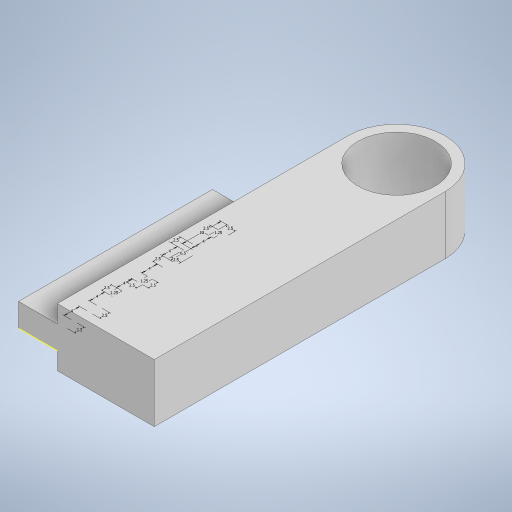
# Autodesk Inventor part: Part10
Saved by Autodesk Inventor 2023 (Build 270158000, 158)
## iProperties
Created: 2024-11-26
Part Number: Part10
Material: Generic
Document SubType Name: Modeling
Designer: 1ZHUSAM
Density: 1 g/cm^3
Appearance: Default
Author: 1ZHUSAM
Autodesk Inventor part; units mm, degrees
ref_plane "YZ Plane" through (0, 0, 0) normal (1, 0, 0) x (0, 1, 0)
ref_plane "XZ Plane" through (0, 0, 0) normal (0, 1, 0) x (-1, 0, 0)
ref_plane "XY Plane" through (0, 0, 0) normal (0, 0, 1) x (1, 0, 0)
sketch "Sketch1" plane through (0, 0, 0) normal (0, 1, 0) x (-1, 0, 0)
  circle A0 centre (0, 0) radius 10
  circle A1 centre (0, 0) radius 12.5
  line L0 (12.5, 0) -> (12.5, 50)
  line L1 (-12.5, 0) -> (-12.5, 50)
  line L2 (-12.5, 50) -> (12.5, 50)
  dimension "d0" = 20
  dimension "d1" = 25
  dimension "d2" = 50
  constraints: 6 end point, 2 centre point, 2 coincident, 2 point on circle, 2 tangent, 2 vertical, 1 perpendicular
  measures "d0" diameter of A0
  measures "d1" diameter of A1
  measures "d2" distance of L0.start L0.end
extrude "Extrusion1" add sketch "Sketch1" along normal blind 15
sketch "Sketch2" plane through (-12.5, 0, 0) normal (-1, 0, 0) x (0, 0, 1)
  line L0 (-12.5, 0) -> (-12.5, 15) projected
  line L1 (-12.5, 7.5) -> (37.5, 7.5)
  line L2 (25, 7.5) -> (25, 4.5)
  line L3 (25, 4.5) -> (25, 10.5)
  line L4 (25, 10.5) -> (75, 10.5)
  line L5 (75, 10.5) -> (75, 4.5)
  line L6 (75, 4.5) -> (25, 4.5)
  point P0 (0, 0)
  dimension "d5" = 50
  dimension "d8" = 3
  dimension "d9" = 6
  dimension "d10" = 50
  constraints: 12 end point, 3 perpendicular, 2 horizontal, 2 point on line, 1 midpoint
  measures "d5" distance of L1.start L1.end
  measures "d8" distance of L2.start L2.end
  measures "d9" distance of L2.end L3.end
  measures "d10" distance of L3.end L4.end
extrude "Extrusion2" add sketch "Sketch2" along normal blind 10
sketch "Sketch3" plane through (-12.5, 0, 50) normal (0, 0, 1) x (1, 0, 0)
  point P0 (12.5, 0)
sketch "Sketch4" plane through (-12.5, 0, 50) normal (0, 0, 1) x (1, 0, 0)
  line L0 (25, 0) -> (25, 15) projected
  line L1 (25, 0) -> (25, 15)
  line L2 (0, 15) -> (25, 15) projected
  line L3 (25, 15) -> (0, 15)
  line L4 (0, 0) -> (0, 15) projected
  line L5 (0, 15) -> (0, 0)
  line L6 (0, 0) -> (25, 0) projected
  line L7 (0, 0) -> (25, 0)
  point P0 (12.5, 0)
  constraints: 8 end point, 4 collinear
extrude "Extrusion3" add sketch "Sketch4" along normal blind 25
sketch "Sketch5" plane through (-12.5, 4.5, 25) normal (0, -1, 0) x (1, 0, 0)
  point P0 (12.5, -25)
sketch "Sketch6" plane through (-12.5, 4.5, 25) normal (0, -1, 0) x (1, 0, 0)
  line L0 (0, 0) -> (-10, 0) projected
  line L1 (-5, 0) -> (-5, 50)
  line L2 (0, 50) -> (-10, 50) projected
  line L3 (-5, 0) -> (-5, 10)
  line L4 (-3.75, 8.75) -> (-6.25, 8.75)
  line L5 (-6.25, 8.75) -> (-6.25, 11.25)
  line L6 (-6.25, 11.25) -> (-3.75, 11.25)
  line L7 (-3.75, 11.25) -> (-3.75, 8.75)
  line L8 (-3.75, 8.75) -> (-6.25, 11.25) construction
  line L9 (-6.25, 8.75) -> (-3.75, 11.25) construction
  line L10 (-5, 11.25) -> (-5, 15.25)
  line L11 (-3.75, 15.25) -> (-6.25, 15.25)
  line L12 (-6.25, 15.25) -> (-6.25, 17.75)
  line L13 (-6.25, 17.75) -> (-3.75, 17.75)
  line L14 (-3.75, 17.75) -> (-3.75, 15.25)
  point P0 (12.5, -25)
  dimension "d15" = 10
  dimension "d16" = 2.5
  dimension "d17" = 2.5
  dimension "d18" = 4
  dimension "d19" = 2.5
  constraints: 26 end point, 5 midpoint, 4 parallel, 2 horizontal, 2 perpendicular, 2 point on line
  measures "d15" distance of L1.start L3.end
  measures "d16" distance of L5.end L6.end
  measures "d17" distance of L4.end L5.end
  measures "d18" distance of L10.start L10.end
  measures "d19" distance of L11.end L12.end
sketch "Sketch7" plane through (-12.5, 4.5, 25) normal (0, -1, 0) x (1, 0, 0)
  line L0 (-4.9925, 17.7874) -> (-4.9925, 21.7874)
  line L1 (-4.9925, 21.7874) -> (-3.7425, 21.7874)
  line L2 (-3.7425, 21.7874) -> (-3.7425, 24.2874)
  line L3 (-3.7425, 24.2874) -> (-6.2425, 24.2874)
  line L4 (-6.2425, 24.2874) -> (-6.2425, 21.7874)
  line L5 (-6.2425, 21.7874) -> (-4.9925, 21.7874)
  line L6 (-4.9925, 24.2874) -> (-4.9925, 28.2874)
  line L7 (-4.9925, 28.2874) -> (-6.2425, 28.2874)
  line L8 (-6.2425, 28.2874) -> (-6.2425, 30.7874)
  line L9 (-6.2425, 30.7874) -> (-3.7425, 30.7874)
  line L10 (-3.7425, 30.7874) -> (-3.7425, 28.2874)
  line L11 (-4.9925, 28.2874) -> (-3.7425, 28.2874)
  line L12 (-4.9925, 30.7874) -> (-4.9925, 34.7874)
  line L13 (-4.9925, 34.7874) -> (-3.7425, 34.7874)
  line L14 (-3.7425, 34.7874) -> (-3.7425, 37.2874)
  line L15 (-3.7425, 37.2874) -> (-6.2425, 37.2874)
  line L16 (-6.2425, 37.2874) -> (-6.2425, 34.7874)
  line L17 (-6.2425, 34.7874) -> (-4.9925, 34.7874)
  line L18 (-4.9925, 37.2874) -> (-4.9925, 41.2874)
  line L19 (-4.9925, 41.2874) -> (-3.7425, 41.2874)
  line L20 (-3.7425, 41.2874) -> (-3.7425, 43.7874)
  line L21 (-3.7425, 43.7874) -> (-6.2425, 43.7874)
  line L22 (-6.2425, 43.7874) -> (-6.2425, 41.2874)
  line L23 (-6.2425, 41.2874) -> (-4.9925, 41.2874)
  line L24 (-5, 15.2622) -> (-5, 8.7622)
  line L25 (-5, 8.7622) -> (-5, 4.7622)
  line L26 (-5, 4.7622) -> (-6.25, 4.7622)
  line L27 (-6.25, 4.7622) -> (-6.25, 2.2622)
  line L28 (-6.25, 2.2622) -> (-3.75, 2.2622)
  line L29 (-3.75, 2.2622) -> (-3.75, 4.7622)
  line L30 (-3.75, 4.7622) -> (-5, 4.7622)
  point P0 (12.5, -25)
  dimension "d20" = 4
  dimension "d21" = 1.25
  dimension "d22" = 2.5
  dimension "d23" = 2.5
  dimension "d24" = 4
  dimension "d25" = 1.25
  dimension "d26" = 2.5
  dimension "d27" = 4
  dimension "d28" = 2.5
  dimension "d29" = 4
  dimension "d30" = 2.5
  dimension "d31" = 6.5
  dimension "d32" = 4
  dimension "d33" = 1.25
  dimension "d34" = 2.5
  dimension "d35" = 2.5
  constraints: 62 end point, 18 perpendicular, 11 point on line, 4 vertical, 3 midpoint, 2 horizontal, 1 collinear
  measures "d20" distance of L0.start L0.end
  measures "d21" distance of L0.end L1.end
  measures "d22" distance of L1.end L2.end
  measures "d23" distance of L2.end L3.end
  measures "d24" distance of L6.start L6.end
  measures "d25" distance of L6.end L7.end
  measures "d26" distance of L7.end L8.end
  measures "d27" distance of L12.start L12.end
  measures "d28" distance of L13.end L14.end
  measures "d29" distance of L18.start L18.end
  measures "d30" distance of L19.end L20.end
  measures "d31" distance of L24.start L24.end
  measures "d32" distance of L24.end L25.end
  measures "d33" distance of L25.end L26.end
  measures "d34" distance of L26.end L27.end
  measures "d35" distance of L27.end L28.end
body "Solid1"
